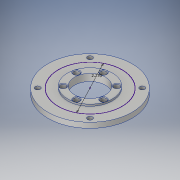
# Autodesk Inventor part: heatsink
Saved by Autodesk Inventor 2018 (Build 220112000, 112)
## iProperties
Created: 2019-03-04
Part Number: heatsink
Material: Aluminum 6061
Document SubType Name: Modeling
Designer: Admin
Density: 2.7 g/cm^3
Appearance: Aluminum - Flat
Author: Admin
Autodesk Inventor part; units mm, degrees
ref_plane "YZ Plane" through (0, 0, 0) normal (1, 0, 0) x (0, 1, 0)
ref_plane "XZ Plane" through (0, 0, 0) normal (0, 1, 0) x (-1, 0, 0)
ref_plane "XY Plane" through (0, 0, 0) normal (0, 0, 1) x (1, 0, 0)
sketch "Sketch1" plane through (0, 0, 0) normal (0, 1, 0) x (-1, 0, 0)
  circle A0 centre (0, 0) radius 13.97
  circle A1 centre (0, 0) radius 38.1
  dimension "d0" = 27.94
  dimension "d1" = 76.2
  constraints: 2 centre point, 2 coincident
  measures "d0" diameter of A0
  measures "d1" diameter of A1
extrude "Extrusion1" add sketch "Sketch1" along normal blind 6.35
sketch "Sketch2" plane through (0, 6.35, 0) normal (0, 1, 0) x (1, 0, 0)
  circle A0 centre (0, 0) radius 20.32
  circle A1 centre (0, 0) radius 13.97 projected
  circle A2 centre (0, 0) radius 38.1
  circle A3 centre (0, 0) radius 38.1 projected
  dimension "d4" = 6.35
  constraints: 2 centre point, 2 coincident, 1 concentric
  measures "d4" radial gap between concentric circles of A0 A1
extrude "Extrusion2" cut sketch "Sketch2" against normal blind 1.5875 contours A2
sketch "Sketch3" plane through (0, 6.35, 0) normal (0, 1, 0) x (1, 0, 0)
  line L0 (0, 0) -> (12.2131, 12.2131) construction
  line L1 (0, 0) -> (17.272, 0) construction
  dimension "d7" = 17.272
  dimension "d8" = 45
  constraints: 4 end point, 1 coincident, 1 equal length, 1 horizontal
  measures "d7" distance of L0.start L0.end
  measures "d8" angle of L1 L0
hole "Hole1" at (12.2131, 6.35, -12.2131) direction (0, -1, 0) diameter 5.1054 depth 25.4 tip angle 118 clearance for "Flat Head Machine Screw (82)" size "#10" standard "Ansi Unified Screw Threads"
chamfer "Chamfer1" distance 0.508 angle 45 2 edges at (12.2131, 6.35, -14.7658) (12.2131, 0, -14.7658)
pattern_circular "Circular Pattern1" count 6 over 360 about axis through (0, 0, 0) along (0, 1, 0) of "Hole1", "Chamfer1"
sketch "Sketch5" plane through (0, 4.7625, 0) normal (0, 1, 0) x (1, 0, 0)
  circle A0 centre (0, 0) radius 28.829
  dimension "d31" = 57.658
  constraints: 1 centre point, 1 coincident
  measures "d31" diameter of A0
sketch "Sketch4" plane through (0, 4.7625, 0) normal (0, 1, 0) x (1, 0, 0)
  circle A0 centre (0, 0) radius 33.528
  circle A1 centre (0, 0) radius 38.1 projected
  line L0 (23.7079, -23.7079) -> (-23.7079, -23.7079)
  line L1 (-23.7079, -23.7079) -> (-23.7079, 23.7079)
  line L2 (-23.7079, 23.7079) -> (23.7079, 23.7079)
  line L3 (23.7079, 23.7079) -> (23.7079, -23.7079)
  line L4 (23.7079, -23.7079) -> (-23.7079, 23.7079) construction
  line L5 (-23.7079, -23.7079) -> (23.7079, 23.7079) construction
  dimension "d32" = 4.572
  constraints: 12 end point, 5 coincident, 2 midpoint, 2 parallel, 1 horizontal, 1 perpendicular, 4 other
hole "Hole2" at (-23.7079, 4.7625, 23.7079) at (23.7079, 4.7625, 23.7079) at (23.7079, 4.7625, -23.7079) at (-23.7079, 4.7625, -23.7079) direction (0, -1, 0) diameter 4.4958 depth 25.4 tip angle 118 clearance for "Flat Head Machine Screw (82)" size "#8" standard "Ansi Unified Screw Threads"
body "Solid1"
